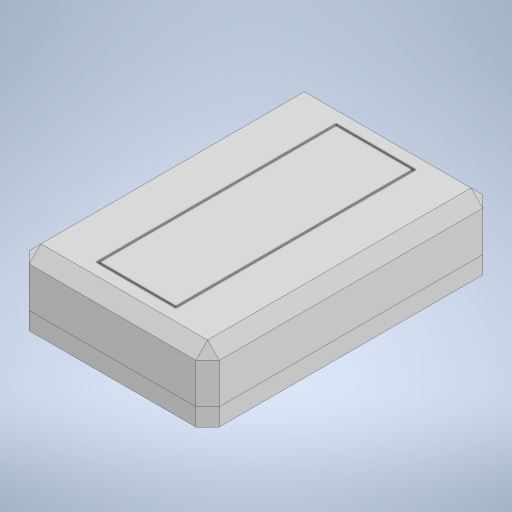
# Autodesk Inventor part: display badge
Saved by Autodesk Inventor 2024 (Build 280153020, 153B)
## iProperties
Created: 2023-08-09
Part Number: display badge
Material: Generic
Document SubType Name: Modeling
Designer: torban
Density: 1 g/cm^3
Appearance: Default
Author: torban
Autodesk Inventor part; units mm, degrees
ref_plane "YZ Plane" through (0, 0, 0) normal (1, 0, 0) x (0, 1, 0)
ref_plane "XZ Plane" through (0, 0, 0) normal (0, 1, 0) x (-1, 0, 0)
ref_plane "XY Plane" through (0, 0, 0) normal (0, 0, 1) x (1, 0, 0)
sketch "Sketch1" plane through (0, 0, 0) normal (0, 1, 0) x (-1, 0, 0)
  line L0 (0, 0) -> (13, 0)
  line L1 (13, 0) -> (13, -40.3)
  line L2 (13, -40.3) -> (0, -40.3)
  line L3 (0, -40.3) -> (0, 0)
  dimension "d0" = 13
  dimension "d1" = 40.3
  constraints: 8 end point, 2 parallel, 1 horizontal, 1 perpendicular
  measures "d0" distance of L1.end L2.end
  measures "d1" distance of L0.end L1.end
extrude "Extrusion1" add sketch "Sketch1" along normal blind 7
sketch "Sketch2" plane through (0, 0, 0) normal (0, -1, 0) x (1, 0, 0)
  line L0 (0, -40.3) -> (-13, -40.3) projected
  line L1 (0, 0) -> (0, -40.3) projected
  line L2 (-13, 0) -> (0, 0) projected
  line L3 (-13, -40.3) -> (-13, 0) projected
  line L4 (-13, 0) -> (0, 0) projected
  line L5 (-13, 0) -> (-18.4, 0)
  line L6 (-18.4, 0) -> (-18.4, -40.3)
  line L7 (-18.4, -40.3) -> (-13, -40.3)
  line L8 (-13, -40.3) -> (-13, 0)
  line L9 (0, 0) -> (5.4, 0)
  line L10 (5.4, 0) -> (5.4, -40.3)
  line L11 (5.4, -40.3) -> (0, -40.3)
  line L12 (0, -40.3) -> (0, 0)
  dimension "d4" = 40.3
  dimension "d5" = 5.4
  dimension "d6" = 5.4
  constraints: 16 end point, 4 parallel, 2 horizontal, 2 perpendicular, 1 point on line
  measures "d4" distance of L9.end L10.end
  measures "d5" distance between parallel lines of L3 L6
  measures "d6" distance of L4.end L9.end
extrude "Extrusion2" add sketch "Sketch2" along normal blind 1.85
sketch "Sketch3" plane through (0, 0, 0) normal (0, 1, 0) x (1, 0, 0)
  line L0 (0, 0) -> (0, 40.3) projected
  line L1 (5.4, 0) -> (0, 0) projected
  line L2 (5.4, 40.3) -> (5.4, 0) projected
  line L3 (0, 40.3) -> (5.4, 40.3) projected
  line L4 (-13, 40.3) -> (-13, 0) projected
  line L5 (-18.4, 40.3) -> (-13, 40.3) projected
  line L6 (-18.4, 0) -> (-18.4, 40.3) projected
  line L7 (-13, 0) -> (-18.4, 0) projected
  line L8 (5.4, 3) -> (0, 3)
  line L9 (0, 3) -> (0, -3)
  line L10 (0, -3) -> (5.4, -3)
  line L11 (5.4, -3) -> (5.4, 3)
  line L12 (-18.4, 3) -> (-13, 3)
  line L13 (-13, 3) -> (-13, -3)
  line L14 (-13, -3) -> (-18.4, -3)
  line L15 (-18.4, -3) -> (-18.4, 3)
  point P0 (0, 3)
  dimension "d9" = 3
  dimension "d10" = 3
  dimension "d11" = 3
  dimension "d12" = 3
  dimension "d13" = 13
  dimension "d14" = 5.4
  dimension "d15" = 5.4
  constraints: 16 end point, 4 parallel, 2 horizontal, 2 perpendicular, 2 point on line
  measures "d9" distance between parallel lines of L7 L12
  measures "d10" distance between parallel lines of L1 L8
  measures "d11" distance between parallel lines of L10 L1
  measures "d12" distance between parallel lines of L14 L7
  measures "d13" distance between parallel lines of L9 L13
  measures "d14" distance between parallel lines of L11 L9
  measures "d15" distance between parallel lines of L15 L13
extrude "Extrusion3" add sketch "Sketch3" along normal blind 1.85 contours L0 L8 L2 L1 | L1 L11 L10 L9 | L4 L7 L6 L12 | L13 L14 L15 L7
sketch "Sketch4" plane through (0, 0, 0) normal (0, 1, 0) x (1, 0, 0)
  line L0 (0, 40.3) -> (-13, 40.3) projected
  line L1 (-13, 40.3) -> (-13, 0) projected
  line L2 (-13, 0) -> (0, 0) projected
  line L3 (0, 0) -> (0, 40.3) projected
  line L4 (0, 3) -> (5.4, 3) projected
  line L5 (5.4, 40.3) -> (5.4, 3) projected
  line L6 (0, 40.3) -> (5.4, 40.3) projected
  line L7 (0, 3) -> (0, 40.3) projected
  line L8 (-18.4, 3) -> (-13, 3) projected
  line L9 (-13, 40.3) -> (-13, 3) projected
  line L10 (-18.4, 40.3) -> (-13, 40.3) projected
  line L11 (-18.4, 3) -> (-18.4, 40.3) projected
  line L12 (0, 40.3) -> (5.4, 40.3) projected
  line L13 (-18.4, 0) -> (-18.4, 40.3) projected
  line L14 (5.4, 40.3) -> (-18.4, 40.3)
  line L15 (-18.4, 40.3) -> (-18.4, 0)
  line L16 (-18.4, 0) -> (5.4, 0)
  line L17 (5.4, 0) -> (5.4, 40.3)
  line L18 (5.7, 40.6) -> (-18.7, 40.6)
  line L19 (-18.7, 40.6) -> (-18.7, -0.3)
  line L20 (-18.7, -0.3) -> (5.7, -0.3)
  line L21 (5.7, -0.3) -> (5.7, 40.6)
  line L22 (0.3, 40) -> (5.1, 40)
  line L23 (5.1, 40) -> (5.1, 3.3)
  line L24 (5.1, 3.3) -> (0.3, 3.3)
  line L25 (0.3, 3.3) -> (0.3, 40)
  line L26 (-13.3, -0.3) -> (-13.3, 40.6)
  line L27 (-13.3, 40.6) -> (0.3, 40.6)
  line L28 (0.3, 40.6) -> (0.3, -0.3)
  line L29 (0.3, -0.3) -> (-13.3, -0.3)
  line L30 (9.7, 44.6) -> (-22.7, 44.6)
  line L31 (-22.7, 44.6) -> (-22.7, -4.3)
  line L32 (-22.7, -4.3) -> (9.7, -4.3)
  line L33 (9.7, -4.3) -> (9.7, 44.6)
  point P0 (0.3, 40.6)
  point P1 (0.3, 3.3)
  point P2 (0.3, 3)
  point P3 (0.3, 0)
  point P4 (0.3, -0.3)
  point P5 (-13.3, 0)
  point P6 (-13.3, 3)
  dimension "d18" = 0.3
  dimension "d19" = 0.3
  dimension "d20" = 0.3
  dimension "d21" = 4
  constraints: 40 end point, 6 parallel, 3 perpendicular, 1 horizontal, 12 other
  measures "d18" distance between parallel lines of L17 L21
  measures "d19" distance between parallel lines of L7 L25
  measures "d20" distance between parallel lines of L1 L26
  measures "d21" distance between parallel lines of L21 L33
extrude "Extrusion4" add sketch "Sketch4" along normal up to surface (7 mm away) separate body contours L28 L18 L21 L20 L16 L17 L5 L6 | L6 L5 L4 L28 L24 L23 L22 | L26 L8 L11 L10 | L10 L11 L13 L16 L26 L20 L19 L18 | L22 L23 L24 L25 | L33 L32 L31 L30
sketch "Sketch5" plane through (-22.7, 7, -44.6) normal (0, 1, 0) x (1, 0, 0)
  line L0 (22.7, -4.3) -> (22.7, -44.6) projected
  line L1 (22.7, -44.6) -> (9.7, -44.6) projected
  line L2 (9.7, -44.6) -> (9.7, -4.3) projected
  line L3 (9.7, -4.3) -> (22.7, -4.3) projected
  line L4 (9.4, -4) -> (9.4, -41.6) projected
  line L5 (9.4, -41.6) -> (4.3, -41.6) projected
  line L6 (4.3, -41.6) -> (4.3, -44.6) projected
  line L7 (4.3, -44.6) -> (9.4, -44.6) projected
  line L8 (9.4, -44.6) -> (9.4, -44.9) projected
  line L9 (9.4, -44.9) -> (23, -44.9) projected
  line L10 (23, -44.9) -> (23, -44.6) projected
  line L11 (23, -44.6) -> (28.1, -44.6) projected
  line L12 (28.1, -44.6) -> (28.1, -41.6) projected
  line L13 (28.1, -41.6) -> (23, -41.6) projected
  line L14 (23, -41.6) -> (23, -4) projected
  line L15 (23, -4) -> (9.4, -4) projected
  line L16 (0, 0) -> (32.4, 0) projected
  line L17 (32.4, 0) -> (32.4, -48.9) projected
  line L18 (32.4, -48.9) -> (0, -48.9) projected
  line L19 (0, -48.9) -> (0, 0) projected
  line L20 (28.1, -41.6) -> (23, -41.6)
  line L21 (23, -41.6) -> (23, -44.6)
  line L22 (23, -44.6) -> (28.1, -44.6)
  line L23 (28.1, -44.6) -> (28.1, -41.6)
  line L24 (4.3, -41.6) -> (9.4, -41.6)
  line L25 (9.4, -41.6) -> (9.4, -44.6)
  line L26 (9.4, -44.6) -> (4.3, -44.6)
  line L27 (4.3, -44.6) -> (4.3, -41.6)
  constraints: 16 end point, 4 parallel, 2 horizontal, 2 perpendicular
extrude "Extrusion5" add sketch "Sketch5" against normal up to surface (5.15 mm away) contours L25 L7 L6 L5 | L13 L12 L11 L21 | L16 L17 L18 L19 bodies 2
sketch "Sketch6" plane through (0, 0, 0) normal (0, -1, 0) x (1, 0, 0)
  line L0 (-13, 3) -> (-13, 0) projected
  line L1 (-13, 0) -> (-18.4, 0) projected
  line L2 (-18.4, 0) -> (-18.4, 3) projected
  line L3 (-18.4, 3) -> (-13, 3) projected
  line L4 (-13, 0) -> (0, 0) projected
  line L5 (5.4, 0) -> (0, 0) projected
  line L6 (5.4, 3) -> (5.4, 0) projected
  line L7 (0, 3) -> (5.4, 3) projected
  line L8 (0, 0) -> (0, 3) projected
  line L9 (-18.4, -3) -> (-18.4, 0) projected
  line L10 (-18.4, -40.3) -> (-18.4, -3) projected
  line L11 (-13, -40.3) -> (-18.4, -40.3) projected
  line L12 (0, -40.3) -> (-13, -40.3) projected
  line L13 (0, -3) -> (0, -40.3) projected
  line L14 (5.4, -3) -> (0, -3) projected
  line L15 (5.4, 0) -> (5.4, -3) projected
  line L16 (-13, -3) -> (-18.4, -3) projected
  line L17 (-13, -3) -> (-13, -40.3) projected
  line L18 (5.4, -40.3) -> (0, -40.3) projected
  line L19 (5.4, -3) -> (5.4, -40.3) projected
  line L20 (9.7, -44.6) -> (-22.7, -44.6) projected
  line L21 (-22.7, -44.6) -> (-22.7, 4.3) projected
  line L22 (-22.7, 4.3) -> (9.7, 4.3) projected
  line L23 (9.7, 4.3) -> (9.7, -44.6) projected
  line L24 (0.3, 0) -> (0.3, 0.3) projected
  line L25 (0.3, 0.3) -> (-13.3, 0.3) projected
  line L26 (-13.3, 0.3) -> (-13.3, 0) projected
  line L27 (-13.3, 0) -> (-18.4, 0) projected
  line L28 (-18.4, 0) -> (-18.4, -3) projected
  line L29 (-18.4, -3) -> (-13.3, -3) projected
  line L30 (-13.3, -3) -> (-13.3, -40.6) projected
  line L31 (-13.3, -40.6) -> (0.3, -40.6) projected
  line L32 (0.3, -40.6) -> (0.3, -3) projected
  line L33 (0.3, -3) -> (5.4, -3) projected
  line L34 (5.4, -3) -> (5.4, 0) projected
  line L35 (5.4, 0) -> (0.3, 0) projected
  line L36 (5.4, 3) -> (5.4, 0) projected
  line L37 (-18.4, -40.3) -> (5.4, -40.3)
  line L38 (5.4, -40.3) -> (5.4, 0)
  line L39 (5.4, 0) -> (-18.4, 0)
  line L40 (-18.4, 0) -> (-18.4, -40.3)
  line L41 (5.7, 0.3) -> (5.7, -40.6)
  line L42 (5.7, -40.6) -> (-18.7, -40.6)
  line L43 (-18.7, -40.6) -> (-18.7, 0.3)
  line L44 (-18.7, 0.3) -> (5.7, 0.3)
  line L45 (-18.7, 0) -> (-18.7, 3.3)
  line L46 (-18.7, 3.3) -> (-12.7, 3.3)
  line L47 (-12.7, 3.3) -> (-12.7, 0)
  line L48 (0.3, 0) -> (0.3, 2.7)
  line L49 (0.3, 2.7) -> (5.4, 2.7)
  line L50 (5.7, 3) -> (5.7, 0)
  line L51 (5.4, 3) -> (5.4, -3) projected
  line L52 (5.7, 3) -> (5.4, 3)
  point P0 (-18.7, 0.3)
  point P1 (-12.7, 0.3)
  point P2 (0, 0.3)
  dimension "d26" = 0.3
  dimension "d27" = 0.3
  dimension "d28" = 0.3
  dimension "d29" = 0.3
  constraints: 30 end point, 5 parallel, 2 horizontal, 2 perpendicular, 6 other
  measures "d26" distance between parallel lines of L38 L41
  measures "d27" distance between parallel lines of L2 L45
  measures "d28" distance between parallel lines of L8 L48
  measures "d29" distance between parallel lines of L6 L50
extrude "Extrusion6" add sketch "Sketch6" along normal up to surface (1.85 mm away) bodies 2
sketch "Sketch7" plane through (-22.7, -1.85, 4.3) normal (0, -1, 0) x (1, 0, 0)
  line L0 (28.1, -4.3) -> (28.1, -44.6) projected
  line L1 (28.1, -44.6) -> (4.3, -44.6) projected
  line L2 (4.3, -44.6) -> (4.3, -4.3) projected
  line L3 (4.3, -4.3) -> (28.1, -4.3) projected
  line L4 (10, -4) -> (10, -1) projected
  line L5 (10, -1) -> (4, -1) projected
  line L6 (4, -1) -> (4, -44.9) projected
  line L7 (4, -44.9) -> (28.4, -44.9) projected
  line L8 (28.4, -44.9) -> (28.4, -1.3) projected
  line L9 (28.4, -1.3) -> (22.7, -1.3) projected
  line L10 (22.7, -1.3) -> (22.7, -4) projected
  line L11 (22.7, -4) -> (10, -4) projected
  line L12 (32.4, 0) -> (32.4, -48.9) projected
  line L13 (32.4, -48.9) -> (0, -48.9) projected
  line L14 (0, -48.9) -> (0, 0) projected
  line L15 (0, 0) -> (32.4, 0) projected
  line L16 (10, -1) -> (4, -1) projected
  line L17 (28.4, -44.9) -> (28.4, -1.3) projected
  line L18 (10, -1) -> (28.4, -1)
  line L19 (28.4, -1) -> (28.4, -4.3)
  line L20 (28.4, -4.3) -> (10, -4.3)
  line L21 (10, -4.3) -> (10, -1)
  point P0 (22.7, -4.3)
  point P1 (28.4, -1.3)
  dimension "d32" = 44.6
  constraints: 8 end point, 2 parallel, 1 horizontal, 1 perpendicular, 1 point on line
  measures "d32" distance between parallel lines of L13 L20
extrude "Extrusion7" cut sketch "Sketch7" against normal up to surface (1.85 mm away) contours L4 L18 L19 L9 L10 L11 bodies 2
sketch "Sketch9" plane through (-22.7, -1.85, 4.3) normal (0, -1, 0) x (1, 0, 0)
  line L0 (0, -48.9) -> (32.4, -48.9) projected
  line L1 (0, -48.9) -> (32.4, -48.9)
  line L2 (32.4, -48.9) -> (32.4, 0)
  line L3 (32.4, 0) -> (0, 0)
  line L4 (0, 0) -> (0, -48.9)
  line L5 (28.4, -1) -> (4, -1) projected
  line L6 (12.2, -1) -> (20.2, -1)
  line L7 (20.2, -1) -> (20.2, -9)
  line L8 (20.2, -9) -> (12.2, -9)
  line L9 (12.2, -9) -> (12.2, -1)
  point P0 (22.7, -4.3)
  point P1 (16.2, -9)
  point P2 (20.2, -1)
  dimension "d39" = 16.2
  dimension "d40" = 16.2
  dimension "d41" = 8
  dimension "d42" = 8
  constraints: 16 end point, 4 parallel, 2 horizontal, 2 perpendicular, 1 midpoint, 1 point on line
  measures "d39" distance from line of L2 point (16.2, -9)
  measures "d40" distance from line of L4 point (16.2, -9)
  measures "d41" distance of L7.end L8.end
  measures "d42" distance between parallel lines of L5 L8
extrude "Extrusion9" add sketch "Sketch9" along normal blind 3 separate body
chamfer "Chamfer1" distance 2 angle 45 12 edges at (-22.7, 7, -20.15) (-6.5, 7, 4.3) (9.7, 7, -20.15) (-6.5, 7, -44.6) (9.7, 2.575, 4.3) (-22.7, 2.575, 4.3) (-22.7, 2.575, -44.6) (9.7, 2.575, -44.6) (9.7, -3.35, -44.6) (-22.7, -3.35, -44.6) (-22.7, -3.35, 4.3) (9.7, -3.35, 4.3)
sketch "Sketch8" plane through (-22.7, -1.85, 4.3) normal (0, -1, 0) x (1, 0, 0)
  line L0 (28.1, -4.3) -> (28.1, -44.6) projected
  line L1 (28.1, -44.6) -> (4.3, -44.6) projected
  line L2 (4.3, -44.6) -> (4.3, -4.3) projected
  line L3 (4.3, -4.3) -> (28.1, -4.3) projected
  line L4 (28.4, -44.9) -> (28.4, -1) projected
  line L5 (28.4, -1) -> (4, -1) projected
  line L6 (4, -1) -> (4, -44.9) projected
  line L7 (4, -44.9) -> (28.4, -44.9) projected
  line L8 (32.4, 0) -> (32.4, -48.9) projected
  line L9 (32.4, -48.9) -> (0, -48.9) projected
  line L10 (0, -48.9) -> (0, 0) projected
  line L11 (0, 0) -> (32.4, 0) projected
  line L12 (4.3, -1.3) -> (9.7, -1.3) projected
  line L13 (22.7, -4.3) -> (22.7, -44.6) projected
  line L14 (9.7, -1.3) -> (22.7, -1.3)
  line L15 (22.7, -1.3) -> (22.7, -6.3)
  line L16 (22.7, -6.3) -> (9.7, -6.3)
  line L17 (9.7, -6.3) -> (9.7, -1.3)
  dimension "d37" = 5
  constraints: 8 end point, 2 parallel, 1 horizontal, 1 perpendicular, 1 point on line
  measures "d37" distance between parallel lines of L14 L16
equation "\"d6\" = d5"
equation "\"d11\" = d10"
equation "\"d12\" = d9"
equation "\"d40\" = d39"
body "Solid1"
